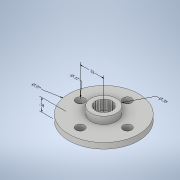
# Autodesk Inventor part: Horn
Saved by Autodesk Inventor 2022 (Build 260153000, 153)
## iProperties
Created: 2019-12-31
Part Number: Horn
Material: Generic
Document SubType Name: Modeling
Designer: KappaCat
Density: 1 g/cm^3
Appearance: Default
Author: KappaCat
Autodesk Inventor part; units mm, degrees
ref_plane "YZ Plane" through (0, 0, 0) normal (1, 0, 0) x (0, 1, 0)
ref_plane "XZ Plane" through (0, 0, 0) normal (0, 1, 0) x (-1, 0, 0)
ref_plane "XY Plane" through (0, 0, 0) normal (0, 0, 1) x (1, 0, 0)
sketch "Sketch1" plane through (0, 0, 0) normal (0, 1, 0) x (-1, 0, 0)
  circle A0 centre (0, 0) radius 12.3
  circle A1 centre (0, 0) radius 4.5
  circle A2 centre (0, 0) radius 2.75
  circle A3 centre (0, 0) radius 1.5
  dimension "d0" = 24.6
  dimension "d1" = 9
  dimension "d2" = 5.5
  dimension "d3" = 3
  constraints: 4 centre point, 4 coincident
  measures "d0" diameter of A0
  measures "d1" diameter of A1
  measures "d2" diameter of A2
  measures "d3" diameter of A3
extrude "Extrusion1" add sketch "Sketch1" along normal blind 2 contours A0
sketch "Sketch2" plane through (0, 0, 0) normal (0, -1, 0) x (1, 0, 0)
  circle A0 centre (0, 0) radius 10
  circle A1 centre (0, 0) radius 4.5
  circle A2 centre (0, 0) radius 2.75
  circle A3 centre (0, 0) radius 1.5
  dimension "d6" = 20
  dimension "d7" = 9
  dimension "d8" = 5.5
  dimension "d9" = 3
  constraints: 4 centre point, 4 coincident
  measures "d6" diameter of A0
  measures "d7" diameter of A1
  measures "d8" diameter of A2
  measures "d9" diameter of A3
extrude "Extrusion2" add sketch "Sketch2" against normal blind 4.5 contours A1
sketch "Sketch3" plane through (0, 0, 0) normal (0, -1, 0) x (1, 0, 0)
  circle A0 centre (0, 0) radius 10
  circle A1 centre (0, 0) radius 4.5
  circle A2 centre (0, 0) radius 2.75
  circle A3 centre (0, 0) radius 1.5
  dimension "d12" = 20
  dimension "d13" = 9
  dimension "d14" = 5.5
  dimension "d15" = 3
  constraints: 4 centre point, 4 coincident
  measures "d12" diameter of A0
  measures "d13" diameter of A1
  measures "d14" diameter of A2
  measures "d15" diameter of A3
extrude "Extrusion3" add sketch "Sketch3" against normal blind 1 contours A2
sketch "Sketch4" plane through (0, 4.5, 0) normal (0, 1, 0) x (1, 0, 0)
  circle A0 centre (0, 0) radius 8.3 construction
  line L0 (0, 0) -> (0, -8.3) construction
  circle A1 centre (0, -8.3) radius 1.5
  dimension "d18" = 16.6
  dimension "d19" = 3
  constraints: 2 coincident, 2 end point, 1 centre point, 1 vertical, 1 vertical alignment, 2 other
  measures "d19" diameter of A1
extrude "Extrusion4" cut sketch "Sketch4" against normal up to next
pattern_circular "Circular Pattern1" count 4 over 360 about axis through (0, 0, 0) along (0, 1, 0) of "Extrusion4"
sketch "Sketch5" plane through (0, 4.5, 0) normal (0, 1, 0) x (1, 0, 0)
  circle A0 centre (0, 0) radius 1.5 projected
  circle A1 centre (0, 0) radius 3 construction
  line L0 (0, 0) -> (0, -3) construction
  line L1 (0, 0) -> (-0.376, -2.9763) construction
  line L2 (0, 0) -> (-0.7461, -2.9057) construction
  circle A2 centre (0, 0) radius 2.75 projected
  line L3 (0, -2.75) -> (-0.376, -2.9763)
  line L4 (-0.6839, -2.6636) -> (-0.376, -2.9763)
  arc A3 (-0.6839, -2.6636) -> (0, -2.75) centre (0, 0) ccw
  dimension "d25" = 6
  dimension "d26" = 7.2
  dimension "d27" = 14.4
  constraints: 10 end point, 7 point on circle, 2 centre point, 2 point on line, 1 coincident, 1 concentric, 1 vertical
  measures "d25" diameter of A1
  measures "d26" angle of L1 L0
  measures "d27" angle of L0 L2
extrude "Extrusion5" cut sketch "Sketch5" against normal up to surface (3.5 mm away) contours A2 L3 L4
pattern_circular "Circular Pattern2" count 25 over 360 about axis through (0, 0, 0) along (0, 1, 0) of "Extrusion5"
body "Solid1"
